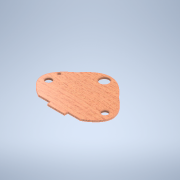
# Autodesk Inventor part: CarTop_V3
Saved by Autodesk Inventor 2022.2 (Build 262287000, 287)
## iProperties
Created: 2022-11-22
Part Number: CarTop_V3
Material: Wood (Oak)
Document SubType Name: Modeling
Designer: jaege
Density: 0.76 g/cm^3
Appearance: Red Oak - Natural Low Gloss
Author: jaege
Autodesk Inventor part; units mm, degrees
ref_plane "YZ Plane" through (0, 0, 0) normal (1, 0, 0) x (0, 1, 0)
ref_plane "XZ Plane" through (0, 0, 0) normal (0, 1, 0) x (-1, 0, 0)
ref_plane "XY Plane" through (0, 0, 0) normal (0, 0, 1) x (1, 0, 0)
sketch "Sketch2" plane through (0, 0, 0) normal (0, 1, 0) x (-1, 0, 0)
  line L0 (-49, 47) -> (-20, 47) construction
  line L1 (49, 47) -> (49, -47) construction
  line L2 (49, -47) -> (-49, -47)
  line L3 (-49, -47) -> (-49, 47) construction
  line L4 (-49, 47) -> (49, -47) construction
  line L5 (49, 47) -> (-49, -47) construction
  line L6 (49, -23) -> (45, -23)
  line L7 (45, -23) -> (45, 27)
  line L8 (45, 27) -> (49, 27)
  line L9 (49, 27) -> (49, -23)
  line L10 (-49, -23) -> (-45, -23)
  line L11 (-45, -23) -> (-45, 27)
  line L12 (-45, 27) -> (-49, 27)
  line L13 (-49, 27) -> (-49, -23)
  line L14 (25, -47) -> (-25, -47)
  line L15 (-25, -47) -> (-25, -43)
  line L16 (-25, -43) -> (25, -43)
  line L17 (25, -43) -> (25, -47)
  line L18 (0, -47) -> (0, 47)
  line L19 (49, 0) -> (-49, 0)
  line L20 (49, 2) -> (-45, 2) construction
  line L21 (20, 47) -> (0, 47) construction
  line L22 (-20, 47) -> (-20, 51) construction
  line L23 (-20, 51) -> (20, 51) construction
  line L24 (20, 51) -> (20, 47) construction
  line L25 (-20, 47) -> (20, 47)
  line L26 (0, 47) -> (-20, 47) construction
  line L27 (20, 47) -> (49, 47) construction
  line L28 (49, 43) -> (20, 43)
  line L29 (20, 43) -> (20, 47)
  line L30 (-49, 43) -> (-20, 43)
  line L31 (-20, 43) -> (-20, 47)
  line L32 (49, 43) -> (49, 27)
  line L33 (-49, 43) -> (-49, 27)
  line L34 (-49, -23) -> (-49, -47)
  line L35 (49, -23) -> (49, -47)
  point P0 (0, 0)
  point P1 (49, 27)
  point P2 (-49, 27)
  point P3 (0, 0)
  point P4 (0, 0)
  dimension "d7" = 98
  dimension "d8" = 94
  dimension "d5" = 4
  dimension "d6" = 50
  dimension "d3" = 4
  dimension "d4" = 50
  dimension "d1" = 50
  dimension "d2" = 4
  dimension "d0" = 2
  dimension "d27" = 4
  dimension "d28" = 40
  dimension "d31" = 4
  constraints: 72 end point, 13 parallel, 12 perpendicular, 9 horizontal, 8 midpoint, 8 point on line, 2 collinear, 1 coincident, 1 horizontal alignment, 3 other
  measures "d7" distance of L1.end L2.end
  measures "d8" distance of L1.start L1.end
  measures "d5" distance of L7.end L8.end
  measures "d6" distance of L6.end L7.end
  measures "d3" distance of L12.end L11.end
  measures "d4" distance of L11.end L10.end
  measures "d1" distance of L15.end L16.end
  measures "d2" distance of L14.end L15.end
  measures "d0" distance between parallel lines of L19 L20
  measures "d27" distance of L0.end L22.end
  measures "d28" distance of L22.end L23.end
  measures "d31" distance from line of L0.start L30
extrude "Extrusion1" add sketch "Sketch2" along normal blind 4 contours L2 L17 L16 L18 L19 L7 L6 L35 | L2 L34 L10 L11 L19 L18 L16 L15 | L19 L18 L25 L29 L28 L32 L8 L7 | L19 L11 L12 L33 L30 L31 L25 L18
sketch "Sketch3" plane through (0, 4, 0) normal (0, 1, 0) x (1, 0, 0)
  circle A0 centre (0, 62.5) radius 11
  spline S0 degree 2 poles (-49, 47) (0, 109) (49, 47) knots 0 0 0 1 1 1
  circle A1 centre (66, -2) radius 7.5
  spline S1 degree 2 poles (49, 47) (117.0544, -3.4606) (49, -43) knots 0 0 0 1 1 1
  line L0 (0, 43) -> (0, -53.479) construction
  circle A2 centre (-66, -2) radius 7.5
  spline S2 degree 2 poles (-49, 47) (-117.0544, -3.4606) (-49, -43) knots 0 0 0 1 1 1
  line L1 (-66, 27) -> (-63.1716, 24.1716)
  line L2 (-63.1716, 24.1716) -> (-67.4142, 19.9289)
  line L3 (-67.4142, 19.9289) -> (-70.2426, 22.7574)
  line L4 (-70.2426, 22.7574) -> (-66, 27)
  line L5 (-20, -47) -> (-20, -51)
  line L6 (-20, -51) -> (20, -51)
  line L7 (20, -51) -> (20, -47)
  line L8 (49, 47) -> (25, 47) construction
  line L9 (25, 47) -> (25, 43) projected
  line L10 (25, 43) -> (-25, 43) projected
  line L11 (-25, 43) -> (-25, 47) projected
  line L12 (-25, 47) -> (-49, 47) construction
  line L13 (-49, 47) -> (-49, 23) construction
  line L14 (-49, 23) -> (-45, 23) projected
  line L15 (-45, 23) -> (-45, -27) projected
  line L16 (-45, -27) -> (-49, -27) projected
  line L17 (-49, -27) -> (-49, -43) construction
  line L18 (-49, -43) -> (-20, -43) projected
  line L19 (-20, -43) -> (-20, -47) projected
  line L20 (-20, -47) -> (20, -47) projected
  line L21 (20, -47) -> (20, -43) projected
  line L22 (20, -43) -> (49, -43) projected
  line L23 (49, -43) -> (49, -27) construction
  line L24 (49, -27) -> (45, -27) projected
  line L25 (45, -27) -> (45, 23) projected
  line L26 (45, 23) -> (49, 23) projected
  line L27 (49, 23) -> (49, 47) construction
  line L28 (-25, 43) -> (-25, 47) projected
  line L29 (-25, 47) -> (25, 47)
  line L30 (49, 23) -> (49, -27)
  line L31 (-49, 47) -> (-49, 23) construction
  line L32 (-49, -27) -> (-49, 23)
  line L33 (-45, 23) -> (-45, -27) construction
  line L34 (-45, -2) -> (45, -2) construction
  point P0 (0, 0)
  point P1 (0, 78)
  point P2 (83, -2)
  point P3 (-83, -2)
  point P4 (-49, -2)
  dimension "d12" = 22
  dimension "d14" = 15.5
  dimension "d18" = 15
  dimension "d19" = 17
  dimension "d21" = 6
  dimension "d22" = 4
  dimension "d29" = 20
  dimension "d33" = 15.5
  dimension "d34" = 17
  dimension "d35" = 4
  dimension "d36" = 45
  dimension "d37" = 17
  constraints: 24 end point, 5 midpoint, 4 perpendicular, 3 centre point, 3 horizontal alignment, 3 vertical, 2 parallel, 2 symmetric about line, 2 vertical alignment, 10 other
  measures "d12" diameter of A0
  measures "d14" distance of A0.centre point (0, 78)
  measures "d18" diameter of A1
  measures "d19" distance of point (83, -2) A1.centre
  measures "d21" distance of L1.end L2.end
  measures "d22" distance of L1.start L1.end
  measures "d29" vertical distance of L12.end L1.start
  measures "d33" distance from line of L29 A0.centre
  measures "d34" distance of point (-49, -2) A2.centre
  measures "d35" distance of L6.end L7.end
  measures "d36" angle of L32 L4
  measures "d37" distance from line of L32 L1.start
extrude "Extrusion2" add sketch "Sketch3" against normal blind 4 contours S0 S1 L22 L21 L20 L19 L18 S2 | L20 L7 L6 L5 | L9 L10 L11 L29 | L14 L15 L16 L32 | L24 L25 L26 L30
body "Solid1"
